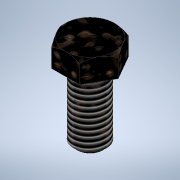
# Autodesk Inventor part: Bolt
Saved by Autodesk Inventor 2020.3 (Build 243373000, 373)
## iProperties
Created: 2021-06-11
Part Number: Bolt
Material: Steel, Mild
Document SubType Name: Modeling
Designer: User
Density: 7.85 g/cm^3
Appearance: Dirt - Dark Brown
Author: User
Autodesk Inventor part; units mm, degrees
ref_plane "YZ Plane" through (0, 0, 0) normal (1, 0, 0) x (0, 1, 0)
ref_plane "XZ Plane" through (0, 0, 0) normal (0, 1, 0) x (-1, 0, 0)
ref_plane "XY Plane" through (0, 0, 0) normal (0, 0, 1) x (1, 0, 0)
sketch "Sketch1" plane through (0, 0, 0) normal (0, 1, 0) x (-1, 0, 0)
  line L0 (8.2561, 0) -> (4.1281, -7.15)
  line L1 (4.1281, -7.15) -> (-4.1281, -7.15)
  line L2 (-4.1281, -7.15) -> (-8.2561, 0)
  line L3 (-8.2561, 0) -> (-4.1281, 7.15)
  line L4 (-4.1281, 7.15) -> (4.1281, 7.15)
  line L5 (4.1281, 7.15) -> (8.2561, 0)
  point P0 (0, 0)
  point P1 (0, 0)
  dimension "d0" = 14.3
  constraints: 12 end point, 1 coincident, 1 horizontal, 13 other
  measures "d0" distance between parallel lines of L1 L4
extrude "Extrusion1" add sketch "Sketch1" along normal blind 6.35
sketch "Sketch2" plane through (0, 6.35, 0) normal (0, 1, 0) x (1, 0, 0)
  circle A0 centre (0, 0) radius 7.15
  dimension "d3" = 14.3
  constraints: 1 centre point, 1 coincident
  measures "d3" diameter of A0
extrude "Extrusion2" cut sketch "Sketch2" against normal through all draft 45 keep common part
sketch "Sketch3" plane through (0, 0, 0) normal (0, -1, 0) x (1, 0, 0)
  circle A0 centre (0, 0) radius 4.765
  dimension "d6" = 9.53
  constraints: 1 centre point, 1 coincident
  measures "d6" diameter of A0
extrude "Extrusion3" add sketch "Sketch3" along normal blind 20.32
chamfer "Chamfer1" distance 1 angle 45 1 edges at (-4.765, -20.32, 0)
fillet "Fillet1" radius 1 1 edges at (-4.765, 0, 0)
thread "Thread1" size "M10x1.5" class "6g" standard "ANSI Metric M Profile" length 18.32
body "Solid1"
